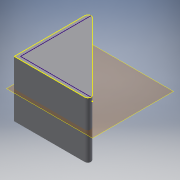
# Autodesk Inventor part: Bracket
Saved by Autodesk Inventor 2019 (Build 230136000, 136)
## iProperties
Created: 2019-04-03
Part Number: Bracket
Material: 일반
Document SubType Name: Modeling
Designer: hinmo
Density: 1 g/cm^3
Appearance: 기본값
Author: hinmo
Autodesk Inventor part; units mm, degrees
ref_plane "YZ Plane" through (0, 0, 0) normal (1, 0, 0) x (0, 1, 0)
ref_plane "XZ Plane" through (0, 0, 0) normal (0, 1, 0) x (-1, 0, 0)
ref_plane "XY Plane" through (0, 0, 0) normal (0, 0, 1) x (1, 0, 0)
sketch "스케치2" plane through (0, 0, 0) normal (0, 1, 0) x (-1, 0, 0)
  line L0 (2.4142, 0) -> (25, 0)
  line L1 (25, 0) -> (25, -22.5858)
  line L2 (23.2929, -23.2929) -> (1.7071, -1.7071)
  arc A0 (23.2929, -23.2929) -> (25, -22.5858) centre (24, -22.5858) ccw
  arc A1 (2.4142, 0) -> (1.7071, -1.7071) centre (2.4142, -1) ccw
  point P0 (0, 0)
  point P1 (25, -25)
  dimension "d2" = 25
  dimension "d3" = 25
  dimension "d4" = 1
  constraints: 6 end point, 4 point on circle, 4 point on line, 4 tangent, 2 centre point, 1 equal radius, 1 horizontal, 1 perpendicular
  measures "d2" distance of point (0, 0) L0.end
  measures "d3" distance of L0.end point (25, -25)
  measures "d4" radius of A0
extrude "돌출1" add sketch "스케치2" along normal blind 18
ref_plane "작업 평면1" through (0, 9, 0) normal (0, 1, 0) x (1, 0, 0)
sketch "스케치4" plane through (0, 18, 0) normal (0, 1, 0) x (1, 0, 0)
  line L0 (-25, 0) -> (-2.4142, 0) projected
  arc A0 (-2.4142, 0) -> (-1.7071, 1.7071) centre (-2.4142, 1) ccw projected
  line L1 (-1.7071, 1.7071) -> (-23.2929, 23.2929) projected
  arc A1 (-23.2929, 23.2929) -> (-25, 22.5858) centre (-24, 22.5858) ccw projected
  line L2 (-25, 22.5858) -> (-25, 0) projected
  line L3 (-24, 22.5858) -> (-24, 1)
  line L4 (-25, 0) -> (-2.4142, 0) projected
  line L5 (-2.4142, 1) -> (-24, 1)
  line L6 (-24, 22.5858) -> (-24, 23.5858)
  line L7 (-2.4142, 1) -> (-1.4142, 1)
  point P0 (0, 0)
  constraints: 8 end point, 2 perpendicular, 2 point on circle, 2 point on line
